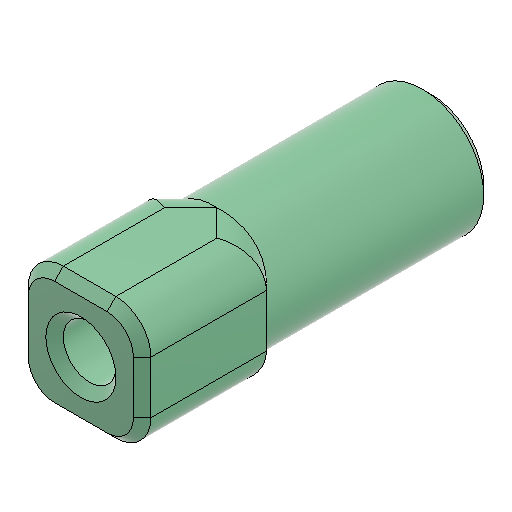
# Autodesk Inventor part: shaft-20mm
Saved by Autodesk Inventor 2026 (Build 300175050, 175E)
## iProperties
Created: 2025-07-16
Part Number: shaft-20mm
Material: ABS Plastic
Document SubType Name: Modeling
Designer: queezz
Density: 1.06 g/cm^3
Appearance: Smooth - Dark Sea Green
Author: queezz
Autodesk Inventor part; units mm, degrees
ref_plane "YZ Plane" through (0, 0, 0) normal (1, 0, 0) x (0, 1, 0)
ref_plane "XZ Plane" through (0, 0, 0) normal (0, 1, 0) x (-1, 0, 0)
sketch "Sketch1" plane through (0, 0, 0) normal (0, 0, 1) x (1, 0, 0)
  circle A0 centre (0, 0) radius 3.5
  circle A1 centre (0, 0) radius 1.5
  dimension "d0" = 3
  dimension "d1" = 7
  constraints: 2 centre point, 2 coincident
  measures "d0" diameter of A1
  measures "d1" diameter of A0
extrude "Extrusion1" add sketch "Sketch1" along normal blind 20
chamfer "Chamfer1" distance 0.5 angle 45 3 edges at (-1.5, 0, 20) (-3.5, 0, 0) (-1.5, 0, 0)
ref_plane "Work Plane1" through (0, 0, 12) normal (0, 0, -1) x (-1, 0, 0)
sketch "Sketch3" plane through (0, 0, 12) normal (0, 0, -1) x (-1, 0, 0)
  line L0 (3.5, 3.5) -> (-3.5, 3.5)
  line L1 (-3.5, 3.5) -> (-3.5, -3.5)
  line L2 (-3.5, -3.5) -> (3.5, -3.5)
  line L3 (3.5, -3.5) -> (3.5, 3.5)
  circle A0 centre (0, 0) radius 3.5 projected
  point P0 (0, 3.5)
  point P1 (3.5, 0)
  point P2 (0, -3.5)
  point P3 (-3.5, 0)
  constraints: 8 end point, 4 tangent, 2 parallel, 1 horizontal, 1 perpendicular
extrude "Extrusion2" add sketch "Sketch3" along normal mid plane 5 contours L3 A0 L0 | A0 L1 L0 | L3 L2 A0 | A0 L2 L1
chamfer "Chamfer2" distance 3.4 angle 45 4 edges at (3.5, 1.75, 9.5) (3.5, -1.75, 9.5) (-3.5, -1.75, 9.5) (-3.5, 1.75, 9.5)
fillet "Fillet2" radius 2 8 edges at (-3.5, 3.5, 13.7) (-3.5, -3.5, 13.7) (3.5, -3.5, 13.7) (3.5, 3.5, 13.7) (1.8, 3.5, 11.2) (-1.8, 3.5, 11.2) (-1.8, -3.5, 11.2) (1.8, -3.5, 11.2)
sketch "Sketch4" plane through (0, 0, 14.5) normal (0, 0, 1) x (1, 0, 0)
  arc A0 (3.5, 1.5) -> (1.5, 3.5) centre (1.5, 1.5) ccw projected
  line L0 (1.5, 3.5) -> (0, 3.5) projected
  arc A1 (3.5, 0) -> (0, 3.5) centre (0, 0) ccw projected
  line L1 (3.5, 0) -> (3.5, 1.5) projected
  arc A2 (1.5, -3.5) -> (3.5, -1.5) centre (1.5, -1.5) ccw projected
  line L2 (3.5, -1.5) -> (3.5, 0) projected
  arc A3 (0, -3.5) -> (3.5, 0) centre (0, 0) ccw projected
  line L3 (0, -3.5) -> (1.5, -3.5) projected
  arc A4 (-3.5, -1.5) -> (-1.5, -3.5) centre (-1.5, -1.5) ccw projected
  line L4 (-1.5, -3.5) -> (0, -3.5) projected
  arc A5 (-3.5, 0) -> (0, -3.5) centre (0, 0) ccw projected
  line L5 (-3.5, 0) -> (-3.5, -1.5) projected
  arc A6 (-1.5, 3.5) -> (-3.5, 1.5) centre (-1.5, 1.5) ccw projected
  line L6 (-3.5, 1.5) -> (-3.5, 0) projected
  arc A7 (0, 3.5) -> (-3.5, 0) centre (0, 0) ccw projected
  line L7 (0, 3.5) -> (-1.5, 3.5) projected
  point P0 (0, 3.5)
  point P1 (0, 3.5)
  point P2 (0, 3.5)
  point P3 (0, 3.5)
extrude "Extrusion3" add sketch "Sketch4" along normal up to surface (5.5 mm away) contours L1 A1 L0 A0 | L2 A2 L3 A3 | A7 L6 A6 L7 | L4 A4 L5 A5
chamfer "Chamfer3" distance 0.5 angle 45 8 edges at (2.9142, -2.9142, 20) (0, -3.5, 20) (-2.9142, -2.9142, 20) (-3.5, 0, 20) (-2.9142, 2.9142, 20) (0, 3.5, 20) (2.9142, 2.9142, 20) (3.5, 0, 20)
body "Solid1"
